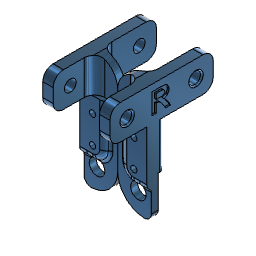
servo_horn_indent_v1.0 (Autodesk Fusion 360 design; units mm, degrees)
Autodesk Fusion 360 part; units mm, degrees
note: some values were not read from the file. Chosen so that the rebuilt part matches the saved one: a direction; that a step has no effect. Set by a fixed rule: which sketch regions a step uses.
sketch "Sketch1" plane through (0, 0, 0) normal (0, 1, 0) x (1, 0, 0) in component "Component"
  circle A0 centre (0, 0) radius 2.25
  line L0 (-6, 6) -> (6, 6)
  line L1 (6, 6) -> (6, -28.6)
  line L2 (6, -28.6) -> (-6, -28.6)
  line L3 (-6, -28.6) -> (-6, 6)
  line L4 (0, 6) -> (0, -28.6) construction
  circle A1 centre (0, -6.1) radius 0.9
  circle A2 centre (0, -6.1) radius 3.5
  circle A3 centre (0, -14.1) radius 0.9
  circle A4 centre (0, -14.1) radius 3.5
  line L5 (3.75, -28.6) -> (3.75, 6)
  line L6 (0, 0) -> (2.25, 0) construction
  line L7 (2.25, 0) -> (2.25, 3.5306) construction
  line L8 (0, -17.6) -> (3.75, -17.6)
  line L9 (0, -10.6) -> (3.75, -10.6)
  line L10 (0, -9.6) -> (3.75, -9.6)
  line L11 (0, -2.6) -> (3.75, -2.6)
  line L12 (-0.25, -28.6) -> (3.75, -28.6)
  line L13 (3.75, -28.6) -> (3.75, -18.6)
  line L14 (3.75, -18.6) -> (-0.25, -18.6)
  line L15 (-0.25, -18.6) -> (-0.25, -28.6)
  line L16 (0, -14.1) -> (-3.5, -14.1) construction
  line L17 (0, -6.1) -> (-3.5, -6.1) construction
  line L18 (-3.5, -6.1) -> (-3.5, -14.1)
  line L19 (-0.25, -18.6) -> (-3.5, -18.6)
  line L20 (-3.5, -14.1) -> (-3.5, -18.6)
  dimension "d1" = 4.5
  dimension "d2" = 12
  dimension "d3" = 6
  dimension "d4" = 6.1
  dimension "d5" = 1.8
  dimension "d6" = 7
  dimension "d7" = 1.8
  dimension "d9" = 7
  dimension "d12" = 1.5
  dimension "d33" = 11
  dimension "d34" = 4
  dimension "d35" = 10
  dimension "d80" = 8
  constraint coincident A0.centre L6.start
  constraint horizontal L0
  constraint vertical L1
  constraint horizontal L2
  constraint vertical L3
  constraint midpoint L0 L4.start
  constraint midpoint L2 L4.end
  constraint coincident A0.centre L4
  constraint coincident L4 A1.centre
  constraint concentric A1 A2
  constraint coincident L4 A3.centre
  constraint concentric A3 A4
  constraint coincident L2 L5.start
  constraint coincident L0 L5.end
  constraint perpendicular L0 L5
  constraint coincident A0 L6.end
  constraint perpendicular L4 L6
  constraint tangent A0 L7
  constraint coincident A4 L8.start
  constraint coincident L4 L8.start
  constraint coincident L5 L8.end
  constraint tangent A4 L8
  constraint coincident A4 L9.start
  constraint coincident L4 L9.start
  constraint coincident L5 L9.end
  constraint tangent A4 L9
  constraint coincident A2 L10.start
  constraint coincident L4 L10.start
  constraint coincident L5 L10.end
  constraint tangent A2 L10
  constraint coincident L4 L11.start
  constraint coincident A2 L11.start
  constraint coincident L5 L11.end
  constraint tangent A2 L11
  constraint horizontal L12
  constraint vertical L13
  constraint horizontal L14
  constraint vertical L15
  constraint coincident L5.start L12.end
  constraint coincident A3.centre A4.centre
  constraint coincident A4 L16.end
  constraint perpendicular L4 L16
  constraint coincident A1.centre A2.centre
  constraint coincident A2 L17.end
  constraint perpendicular L4 L17
  constraint perpendicular L15 L19
  constraint coincident L19 L20.end
  constraint tangent A4 L20
  measures "d1" diameter of A0
  measures "d2" distance of L0.start L0.end
  measures "d3" distance of A0.centre L0
  measures "d4" distance of A0.centre A1.centre
  measures "d5" diameter of A1
  measures "d6" diameter of A2
  measures "d7" diameter of A3
  measures "d9" diameter of A4
  measures "d12" distance of L5 L7
  measures "d33" distance of L2 L8
  measures "d34" distance of L13.end L14.end
  measures "d35" distance of L12.start L14.end
  measures "d80" distance of A1.centre A3.centre
extrude "Extrude3" add sketch "Sketch1" against normal blind 2 contours L0 L2 L3 A2 L5 L11 L15 L18 L19 L20 | A2 L5 L10 L11 | L2 L5 L12 L13 L14 L15 | A2 A4 L5 L9 L10 L18 | A2 | A4 L5 L8 L14 L19 L20 | A4 L5 L8 L9 | A4 makes body 1 in component "Component"
extrude "Extrude4" add sketch "Sketch1" against normal blind 3.3 contours A2 L5 L10 L11 | A2 A4 L5 L9 L10 L18 | A2 | A4 L5 L8 L14 L19 L20 | A4 L5 L8 L9 | A4 bodies 1 in component "Component"
ref_plane "WorkPlane3" through (-1.125, -1, 28.6) normal (0, 0, 1) x (-1, 0, 0) in component "Component"
sketch "Sketch4" plane through (0, 0, 28.6) normal (0, 0, 1) x (1, 0, 0) in component "Component"
  line L0 (3.75, 0) -> (-6, 0)
  line L1 (-6, 0) -> (-6, -2)
  line L2 (-6, -2) -> (3.75, -2)
  line L3 (3.75, -2) -> (3.75, 0)
  line L4 (0.75, 16) -> (3.75, 16)
  line L5 (3.75, 16) -> (3.75, -14)
  line L6 (3.75, -14) -> (0.75, -14)
  line L7 (0.75, -14) -> (0.75, 16)
  line L8 (3.75, 1) -> (0.75, 1) construction
  line L9 (3.75, -1) -> (-6, -1) construction
  dimension "d45" = 3
  dimension "d46" = 30
  dimension "d48" = 2
  constraint horizontal L4
  constraint vertical L5
  constraint horizontal L6
  constraint vertical L7
  constraint midpoint L5 L8.start
  constraint midpoint L7 L8.end
  constraint midpoint L3 L9.start
  constraint midpoint L1 L9.end
  constraint collinear L3 L5
  measures "d45" distance of L5.end L6.end
  measures "d46" distance of L4.start L6.end
  measures "d48" distance of L8 L9
extrude "Extrude7" add sketch "Sketch4" against normal blind 10 contours L0 L2 L3 L5 L7 | L0 L4 L5 L7 | L2 L5 L6 L7 bodies 1 in component "Component"
ref_plane "WorkPlane4" through (3.75, 1, 11.3) normal (1, 0, 0) x (0, 0, 1) in component "Component"
sketch "Sketch5" plane through (3.75, 0, 0) normal (1, 0, 0) x (0, 1, 0) in component "Component"
  line L0 (-3.3, 18.6) -> (-3.3, 2.6)
  line L1 (-3.3, 2.6) -> (-2, 2.6)
  line L2 (-2, 2.6) -> (-2, -6)
  line L3 (-2, -6) -> (0, -6)
  line L4 (0, -6) -> (0, 18.6)
  line L5 (0, 18.6) -> (16, 18.6)
  line L6 (16, 18.6) -> (16, 28.6)
  line L7 (16, 28.6) -> (-14, 28.6)
  line L8 (-14, 28.6) -> (-14, 18.6)
  line L9 (-1.9908, 19.0192) -> (0, 18.6)
  line L10 (-14, 23.6) -> (16, 23.6) construction
  circle A0 centre (11, 23.6) radius 1.7
  line L11 (1, 28.6) -> (1, 18.6) construction
  circle A1 centre (-9, 23.6) radius 1.7
  line L12 (-14, 18.6) -> (-3.3, 18.6)
  dimension "d52" = 3.4
  dimension "d53" = 5
  constraint coincident L4.end L5.start
  constraint midpoint L8 L10.start
  constraint midpoint L6 L10.end
  constraint coincident L10 A0.centre
  constraint midpoint L7 L11.start
  constraint coincident L5 L11.end
  constraint perpendicular L5 L11
  constraint symmetric A0 L11 A1
  measures "d52" diameter of A0
  measures "d53" distance of L6 A0.centre
extrude "Extrude8" cut sketch "Sketch5" against normal up to surface (3 mm away) contours A0 | A1 bodies 1 in component "Component"
ref_plane "WorkPlane5" through (0.75, 8, 23.6) normal (-1, 0, 0) x (0, 1, 0) in component "Component"
sketch "Sketch7" plane through (0.75, 0, 0) normal (-1, 0, 0) x (0, -1, 0) in component "Component"
  circle A0 centre (-11, 23.6) radius 1.7
  circle A1 centre (9, 23.6) radius 1.7
  circle A2 centre (-11, 23.6) radius 4
  circle A3 centre (9, 23.6) radius 4
  dimension "d57" = 8
  dimension "d58" = 8
  constraint concentric A0 A2
  constraint concentric A1 A3
  measures "d57" diameter of A2
  measures "d58" diameter of A3
fillet "Fillet9" radius 8 1 edges at (-6, -1, -6) on bodies 1 in component "Component"
fillet "Fillet10" radius 2 1 edges at (3.75, -1, -6) on bodies 1 in component "Component"
fillet "Fillet11" radius 1.096 3 edges at (1.875, -2, 2.6) (-2.4749, -2, 3.6251) (-3.5, -2, 12.35) on bodies 1 in component "Component"
fillet "Fillet12" radius 2 3 edges at (-3.5, -3.3, 12.35) (-2.4749, -3.3, 3.6251) (1.875, -3.3, 2.6) on bodies 1 in component "Component"
chamfer "Chamfer2" distance 0.4 angle 45 2 edges at (3.75, -10.585, 24.2147) (3.75, 9.415, 24.2147) on bodies 1 in component "Component"
fillet "Fillet15" radius 6 1 edges at (-6, -1, 28.6) on bodies 1 in component "Component"
fillet "Fillet16" radius 3 2 edges at (0.75, -2, 23.6) (0.75, 0, 23.6) on bodies 1 in component "Component"
fillet "Fillet17" [no effect] in component "Component"
fillet "Fillet18" radius 3 4 edges at (2.25, -14, 28.6) (2.25, -14, 18.6) (2.25, 16, 28.6) (2.25, 16, 18.6) on bodies 1 in component "Component"
ref_plane "WorkPlane1" through (-1.125, 0, 11.3) normal (0, 1, 0) x (1, 0, 0)
sketch "Sketch1 (2)" plane through (0, 0, 0) normal (0, 1, 0) x (1, 0, 0)
  circle A0 centre (0, 0) radius 2.25
  circle A1 centre (0, 0) radius 5.3
  line L0 (3.75, -5.3) -> (-6, -5.3)
  circle A2 centre (0, -14.1) radius 0.9
  circle A3 centre (0, -6.1) radius 0.9
  circle A4 centre (0, 0) radius 2.25
  line L1 (-2.25, -28.1621) -> (-2.25, -18.6)
  line L2 (-2.25, -18.6) -> (3.75, -18.6)
  line L3 (3.75, -18.6) -> (3.75, 3.9948)
  arc A5 (3.75, 3.9948) -> (1.6667, 5.9931) centre (1.75, 3.9948) ccw
  arc A6 (1.6667, 5.9931) -> (-6, -2) centre (2, -2) ccw
  line L4 (-6, -2) -> (-6, -22.6)
  arc A7 (-6, -22.6) -> (-2.25, -28.1621) centre (0, -22.6) ccw
  line L5 (3.75, -18.6) -> (-6, -18.6)
  line L6 (-3.82, -19) -> (-3.82, -6.5)
  line L7 (-3.82, -6.5) -> (-3.82, -5.3)
  dimension "d103" = 10.6
  constraint coincident A0.centre A1.centre
  constraint horizontal L0
  constraint tangent A1 L0
  constraint perpendicular L3 L5
  constraint coincident L3 L2.end
  constraint coincident L4 L5.end
  constraint coincident L0.end L4
  constraint coincident L0.start L3
  constraint collinear L2 L5
  constraint coincident L6.end L7.start
  constraint coincident L0 L7.end
  constraint perpendicular L0 L7
  measures "d103" diameter of A1
extrude "Extrude13" add sketch "Sketch1 (2)" along normal blind 1.5 contours L0 A3 L2 L3 L5 L6 L7 bodies 1 in component "Component"
fillet "Fillet19" radius 1 4 edges at (-3.82, 1.5, 11.95) (2.0812, 1.5, 5.3) (-2.1162, 1.5, 5.3) (3.75, 1.5, 11.95) on bodies 1 in component "Component"
ref_plane "WorkPlane2" through (-1.125, 0, 11.3) normal (0, 1, 0) x (1, 0, 0)
sketch "Sketch2" plane through (0, 0, 0) normal (0, 1, 0) x (1, 0, 0)
  line L0 (-5.4198, -20.3089) -> (-2.7706, -20.3089)
  line L1 (-2.7706, -20.3089) -> (-4.0952, -25.5109)
  line L2 (-4.0952, -25.5109) -> (-5.4198, -20.3089)
  constraint horizontal L0
extrude "Extrude14" add sketch "Sketch2" along normal blind 0.5 bodies 1 in component "Component"
mirror "MirrorComponent1" about plane through (0, 0, 0) normal (0, 0, 1) of bodies 1 makes body 2 in component "Component1(Mirror)"
ref_plane "WorkPlane3" through (3.75, 1, 12.3026) normal (1, 0, 0) x (0, 0, 1)
sketch "Sketch3" plane through (3.75, 0, 0) normal (1, 0, 0) x (0, 1, 0)
  line L0 (-1.7478, 19.2484) -> (9.2621, 19.2484) construction
  line L1 (9.2621, 19.2484) -> (9.2621, 26.6664) construction
  line L2 (9.2621, 26.6664) -> (-1.7478, 26.6664) construction
  line L3 (-1.7478, 26.6664) -> (-1.7478, 19.2484) construction
  dimension "d117" = 6
  text T0 "R" font "Arial" height 6 bold align left top in box 11.0099 x 7.418 at (-1.7478, 19.2484) x (1, 0) y (0, 1) spacing 1
extrude "Extrude16" cut sketch "Sketch3" against normal blind 0.5 text T0 bodies 1 in component "Component"
ref_plane "WorkPlane4" through (-15.75, 1, 12.3026) normal (-1, 0, 0) x (0, 0, 1)
sketch "Sketch4 (2)" plane through (-15.75, 0, 0) normal (-1, 0, 0) x (0, -1, 0)
  line L0 (-2.4837, 18.5923) -> (7.9015, 18.5923) construction
  line L1 (7.9015, 18.5923) -> (7.9015, 26.6349) construction
  line L2 (7.9015, 26.6349) -> (-2.4837, 26.6349) construction
  line L3 (-2.4837, 26.6349) -> (-2.4837, 18.5923) construction
  dimension "d121" = 6
  text T0 "L" font "Arial" height 6 bold align left top in box 10.3852 x 8.0427 at (-2.4837, 18.5923) x (1, 0) y (0, 1) spacing 1
extrude "Extrude3'" cut sketch "Sketch4 (2)" against normal blind 0.5 text T0 sketch seen with x (-1, 0, 0) y (0, 1, 0) z (0, 0, -1) at (-12, 0, 0) bodies 2 in component "Component1(Mirror)"
component "Component" placed x (1, 0, 0) y (0, 1, 0) z (0, 0, 1) at (0, 0, 0)
component "Component1(Mirror)" placed x (-1, 0, 0) y (0, 1, 0) z (0, 0, -1) at (-12, 0, 0)
equation "d19 = -4.3 mm + 1.0 mm"
equation "d103 = 5.3 mm * 2"
named bodies: "Body"
